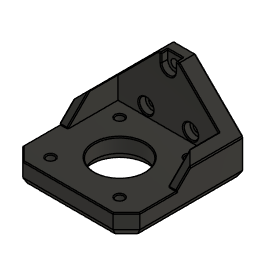
z_axis_bottom_x2 (Autodesk Fusion 360 design; units mm, degrees)
Autodesk Fusion 360 part; units mm, degrees
note: some values were not read from the file. Chosen so that the rebuilt part matches the saved one: which face or edge a step refers to; the sign of a taper; which pieces of a blend or face edit are solid. Set by a fixed rule: which sketch regions a step uses.
sketch "Sketch1" plane through (0, 0, 0) normal (0, 0, 1) x (1, 0, 0)
  line L0 (0, 0) -> (52.5, 0)
  line L1 (52.5, 0) -> (52.5, 52.5)
  line L2 (52.5, 52.5) -> (0, 52.5)
  line L3 (0, 52.5) -> (0, 0)
  line L4 (0, 6) -> (6, 0)
  line L5 (26.25, 0) -> (26.25, 50)
  line L6 (3.7, 22.5) -> (0, 22.5)
  line L7 (3.7, 45) -> (26.25, 45)
  line L8 (3.7, 22.5) -> (3.7, 45)
  circle A0 centre (26.25, 23.2) radius 11.2
  line L9 (48.8, 22.5) -> (52.5, 22.5)
  line L10 (48.8, 22.5) -> (48.8, 45)
  line L11 (48.8, 45) -> (26.25, 45)
  line L12 (52.5, 6) -> (46.5, 0)
  circle A1 centre (10.75, 38.7) radius 1.75
  line L13 (10.75, 38.7) -> (41.75, 7.7) construction
  line L14 (41.75, 38.7) -> (10.75, 7.7) construction
  line L15 (41.75, 38.7) -> (10.75, 38.7) construction
  line L16 (10.75, 38.7) -> (10.75, 7.7) construction
  circle A2 centre (10.75, 38.7) radius 3.25
  line L17 (9, 41.4386) -> (9, 35.9614)
  line L18 (12.5, 41.4386) -> (12.5, 35.9614)
  line L19 (9, 40.45) -> (12.5, 40.45)
  line L20 (12.5, 36.95) -> (9, 36.95)
  line L21 (26.25, 23.2) -> (10.75, 23.2)
  circle A3 centre (10.75, 7.7) radius 3.25
  line L22 (12.5, 9.45) -> (9, 9.45)
  line L23 (12.5, 4.9614) -> (12.5, 10.4386)
  circle A4 centre (10.75, 7.7) radius 1.75
  line L24 (9, 5.95) -> (12.5, 5.95)
  line L25 (9, 4.9614) -> (9, 10.4386)
  line L26 (40, 36.95) -> (43.5, 36.95)
  line L27 (40, 41.4386) -> (40, 35.9614)
  circle A5 centre (41.75, 38.7) radius 1.75
  line L28 (43.5, 40.45) -> (40, 40.45)
  circle A6 centre (41.75, 38.7) radius 3.25
  line L29 (43.5, 41.4386) -> (43.5, 35.9614)
  circle A7 centre (41.75, 7.7) radius 1.75
  line L30 (43.5, 5.95) -> (40, 5.95)
  line L31 (40, 9.45) -> (43.5, 9.45)
  line L32 (40, 4.9614) -> (40, 10.4386)
  line L33 (43.5, 4.9614) -> (43.5, 10.4386)
  circle A8 centre (41.75, 7.7) radius 3.25
  line L34 (3.7, 45) -> (0, 45)
  line L35 (48.8, 45) -> (52.5, 45)
  point P0 (26.25, 23.2)
  dimension "d1" = 52.5
  dimension "d3" = 45
  dimension "d6" = 6
  dimension "d7" = 3.7
  dimension "d8" = 7.5
  dimension "d9" = 22.5
  dimension "d10" = 22.4
  dimension "d11" = 23.2
  dimension "d12" = 3.5
  dimension "d13" = 90
  dimension "d14" = 31
  dimension "d15" = 6.5
  dimension "d65" = 52.5
  constraint horizontal L0
  constraint vertical L1
  constraint horizontal L2
  constraint vertical L3
  constraint coincident L0.start L3.end
  constraint coincident L3 L4.start
  constraint coincident L0 L4.end
  constraint midpoint L0 L5.start
  constraint coincident L3 L6.end
  constraint horizontal L6
  constraint coincident L5 L7.end
  constraint horizontal L7
  constraint vertical L8
  constraint coincident L7.start L8.end
  constraint coincident L5 P0
  constraint symmetric L5 L6.start L9.start
  constraint symmetric L5 L6.end L9.end
  constraint symmetric L5 L7.start L10.end
  constraint symmetric L5 L7.end L11.end
  constraint symmetric L4.start L5 L12.start
  constraint symmetric L4.end L5 L12.end
  constraint midpoint L13 P0
  constraint midpoint P0 L14
  constraint horizontal L15
  constraint coincident A1.centre L13.start
  constraint vertical L16
  constraint coincident L14.end L16.end
  constraint coincident P0 A0.centre
  constraint concentric A1 A2
  constraint coincident A2 L17.start
  constraint coincident A2 L17.end
  constraint coincident A2 L18.start
  constraint coincident A2 L18.end
  constraint vertical L18
  constraint vertical L17
  constraint tangent A1 L17
  constraint tangent A1 L18
  constraint coincident L17 L19.start
  constraint coincident L18 L19.end
  constraint coincident L18 L20.start
  constraint coincident L17 L20.end
  constraint horizontal L19
  constraint horizontal L20
  constraint tangent A1 L19
  constraint tangent A1 L20
  constraint midpoint L16 L21.end
  constraint symmetric A1 L21 A4
  constraint symmetric A2 L21 A3
  constraint symmetric L17.start L21 L25.start
  constraint symmetric L17.end L21 L25.end
  constraint symmetric L18.start L21 L23.start
  constraint symmetric L18.end L21 L23.end
  constraint symmetric L19.start L21 L24.start
  constraint symmetric L19.end L21 L24.end
  constraint symmetric L20.start L21 L22.start
  constraint symmetric L20.end L21 L22.end
  constraint symmetric L5 A1 A5
  constraint symmetric L5 A2 A6
  constraint symmetric L5 L17.start L29.start
  constraint symmetric L5 L17.end L29.end
  constraint symmetric L5 L18.start L27.start
  constraint symmetric L5 L18.end L27.end
  constraint symmetric L5 L19.start L28.start
  constraint symmetric L5 L19.end L28.end
  constraint symmetric L5 L20.start L26.start
  constraint symmetric L5 L20.end L26.end
  constraint vertical L5
  constraint symmetric L5 A3 A8
  constraint symmetric L5 L22.start L31.start
  constraint symmetric L5 L22.end L31.end
  constraint symmetric L5 L23.start L32.start
  constraint symmetric L5 L23.end L32.end
  constraint symmetric L5 A4 A7
  constraint symmetric L5 L24.start L30.start
  constraint symmetric L5 L24.end L30.end
  constraint symmetric L5 L25.start L33.start
  constraint symmetric L5 L25.end L33.end
  constraint coincident L3 L34.end
  constraint perpendicular L3 L34
  constraint symmetric L5 L34.end L35.end
  measures "d1" distance of L0.start L0.end
  measures "d3" angle of L0 L4
  measures "d6" distance of L0.start L4.end
  measures "d7" distance of L6.start L6.end
  measures "d8" distance of L2 L7
  measures "d9" distance of L6.start L7.start
  measures "d10" diameter of A0
  measures "d11" distance of L5.start P0
  measures "d12" diameter of A1
  measures "d13" angle of L13 L14
  measures "d14" distance of L14.start A1.centre
  measures "d15" diameter of A2
  measures "d65" distance of L0.start L2.end
extrude "Extrude1" add sketch "Sketch1" along normal blind 9 contours L0 L3 L4 L5 L6 L7 L8 A0 | L0 L1 L5 A0 L9 L10 L11 L12 | L3 L6 L8 L34 | L1 L9 L10 L35 | A1 L18 L20 | A1 L18 L19 | A2 L18 | A1 L17 L19 | A2 L17 L18 L19 | A1 L17 L20 | A2 L17 L18 L20 | A2 L17 | A3 L23 | A3 L22 L23 L25 | A3 L23 L24 L25 | A3 L25 | L22 L23 A4 | L23 A4 L24 | L22 A4 L25 | A4 L24 L25 | L26 L27 A5 | L26 L27 A6 L29 | L27 A6 | L26 A5 L29 | L27 A5 L28 | A6 L29 | A5 L28 L29 | L27 L28 A6 L29 | A7 L30 L33 | L33 A8 | A7 L31 L33 | A7 L31 L32 | L31 L32 L33 A8 | A7 L30 L32 | L30 L32 L33 A8 | L32 A8
extrude "Extrude2" cut sketch "Sketch1" along normal blind 3.6 contours A1 L18 L20 | A1 L18 L19 | A1 L17 L19 | A1 L17 L20 | L22 L23 A4 | L23 A4 L24 | L22 A4 L25 | A4 L24 L25 | L26 L27 A5 | L26 A5 L29 | L27 A5 L28 | A5 L28 L29 | A7 L30 L33 | A7 L31 L33 | A7 L31 L32 | A7 L30 L32
extrude "Extrude3" cut sketch "Sketch1" along normal blind 3.3 contours A2 L17 L18 L19 | A2 L17 L18 L20 | A3 L22 L23 L25 | A3 L23 L24 L25 | L26 L27 A6 L29 | L27 L28 A6 L29 | L31 L32 L33 A8 | L30 L32 L33 A8
extrude "Extrude4" cut sketch "Sketch1" along normal blind 3 contours A2 L18 | A2 L17 | A3 L23 | A3 L25 | L27 A6 | A6 L29 | L33 A8 | L32 A8
extrude "Extrude6" add sketch "Sketch1" along normal blind 37 contours L1 L2 L3 L7 L11 L34 L35
extrude "Extrude7" add sketch "Sketch1" along normal blind 32 contours L3 L6 L8 L34 | L1 L9 L10 L35
chamfer "Chamfer3" distance 22.5 angle 45 2 edges at (50.65, 22.5, 32) (1.85, 22.5, 32) measured on face at (50.0333, 37.5, 32) measured on face at (1.2333, 37.5, 32)
chamfer "Chamfer4" distance 21.5 angle 45 2 edges at (52.5, 48.75, 37) (0, 48.75, 37) measured on face at (17.5, 50, 37) measured on face at (17.5, 50, 37)
chamfer "Chamfer6" distance 1.5 angle 60 6 edges at (52.5, 29.25, 0) (49.5, 3, 0) (26.25, 0, 0) (3, 3, 0) (0, 29.25, 0) (26.25, 52.5, 0) measured on face at (30.9178, 48.8616, 0) measured on face at (50.5, 4, 3) measured on face at (30.9178, 48.8616, 0) measured on face at (30.9178, 48.8616, 0) measured on face at (30.9178, 48.8616, 0) measured on face at (30.9178, 48.8616, 0)
chamfer "Chamfer7" distance 0.4 angle 45 9 edges at (38.7199, 6.5247, 0) (7.7199, 6.5247, 0) (7.7199, 37.5247, 0) (38.7199, 37.5247, 0) (9.1184, 39.3328, 9) (9.1184, 8.3328, 9) (40.1184, 8.3328, 9) (40.1184, 39.3328, 9) (15.8079, 27.2501, 9) measured on face at (30.9178, 47.8616, 0) measured on face at (30.9178, 47.8616, 0) measured on face at (30.9178, 47.8616, 0) measured on face at (30.9178, 47.8616, 0) measured on face at (42.6306, 28.665, 9) measured on face at (42.6306, 28.665, 9) measured on face at (42.6306, 28.665, 9) measured on face at (42.6306, 28.665, 9) measured on face at (42.6306, 28.665, 9)
chamfer "Chamfer8" distance 1.5 angle 60 1 edges at (15.8079, 19.1499, 0) measured on face at (21.5783, 48.0114, 0)
sketch "Sketch2" plane through (0, 45, 0) normal (0, -1, 0) x (1, 0, 0)
  line L0 (21.5, 37) -> (3.7, 19.2) construction
  line L1 (3.7, 19.2) -> (3.7, 9) construction
  line L2 (3.7, 9) -> (48.8, 9) construction
  line L3 (48.8, 9) -> (48.8, 19.2) construction
  line L4 (48.8, 19.2) -> (31, 37) construction
  line L5 (31, 37) -> (21.5, 37)
  line L6 (26.25, 37) -> (26.25, 9)
  line L7 (3.7, 9) -> (3.7, 0) construction
  line L8 (3.7, 0) -> (48.8, 0) construction
  line L9 (48.8, 0) -> (48.8, 9) construction
  circle A0 centre (16.25, 13) radius 3.25
  circle A1 centre (16.25, 13) radius 1.75
  circle A2 centre (36.25, 13) radius 3.25
  circle A3 centre (36.25, 13) radius 1.75
  circle A4 centre (26.25, 33) radius 3.25
  circle A5 centre (26.25, 33) radius 1.75
  line L10 (23, 33) -> (23, 37)
  line L11 (29.5, 33) -> (29.5, 37)
  line L12 (36.25, 13) -> (16.25, 13) construction
  line L13 (20.25, 8.52) -> (32.25, 8.52)
  line L14 (32.25, 8.52) -> (32.25, 17.48)
  line L15 (32.25, 17.48) -> (20.25, 17.48)
  line L16 (20.25, 17.48) -> (20.25, 8.52)
  line L17 (20.25, 8.52) -> (32.25, 17.48) construction
  line L18 (32.25, 8.52) -> (20.25, 17.48) construction
  line L19 (36.25, 13) -> (46.5, 13) construction
  line L20 (40.25, 8.52) -> (47.5, 8.52)
  line L21 (47.5, 8.52) -> (47.5, 17.48)
  line L22 (47.5, 17.48) -> (40.25, 17.48)
  line L23 (40.25, 17.48) -> (40.25, 8.52)
  line L24 (40.25, 8.52) -> (47.5, 17.48) construction
  line L25 (47.5, 8.52) -> (40.25, 17.48) construction
  line L26 (5, 8.52) -> (5, 17.48)
  line L27 (5, 17.48) -> (12.25, 17.48)
  line L28 (12.25, 17.48) -> (12.25, 8.52)
  line L29 (12.25, 8.52) -> (5, 8.52)
  line L30 (52.5, 2.5981) -> (52.5, 15.5)
  point P0 (26.25, 13)
  point P1 (43.875, 13)
  dimension "d49" = 9
  dimension "d50" = 6.5
  dimension "d51" = 3.5
  dimension "d52" = 20
  dimension "d53" = 13
  dimension "d54" = 6.5
  dimension "d55" = 3.5
  dimension "d56" = 33
  dimension "d68" = 8.96
  dimension "d69" = 4
  dimension "d71" = 8.96
  dimension "d72" = 4
  dimension "d91" = 5
  constraint midpoint L5 L6.start
  constraint midpoint L2 L6.end
  constraint coincident L1.end L2.start
  constraint perpendicular L2 L7
  constraint perpendicular L7 L8
  constraint perpendicular L8 L9
  constraint coincident L2.end L3.start
  constraint concentric A0 A1
  constraint symmetric L6 A0 A2
  constraint symmetric L6 A1 A3
  constraint coincident L6 A4.centre
  constraint concentric A4 A5
  constraint coincident A4 L10.start
  constraint tangent A4 L10
  constraint coincident L5 L10.end
  constraint coincident A4 L11.start
  constraint tangent A4 L11
  constraint coincident L5 L11.end
  constraint vertical L11
  constraint vertical L10
  constraint coincident A2.centre A3.centre
  constraint coincident A0.centre A1.centre
  constraint horizontal L13
  constraint perpendicular L13 L14
  constraint parallel L13 L15
  constraint parallel L14 L16
  constraint coincident L17 P0
  constraint coincident L18 P0
  constraint midpoint L12 P0
  constraint perpendicular L3 L19
  constraint horizontal L20
  constraint perpendicular L20 L21
  constraint parallel L20 L22
  constraint parallel L21 L23
  constraint coincident L24 P1
  constraint coincident L25 P1
  constraint coincident L19 P1
  constraint symmetric L6 L20.start L28.end
  constraint symmetric L6 L20.end L26.start
  constraint symmetric L6 L21.end L26.end
  constraint symmetric L6 L22.end L27.end
  measures "d49" distance of L8.end L2.end
  measures "d50" diameter of A0
  measures "d51" diameter of A1
  measures "d53" distance of L8 A0.centre
  measures "d54" diameter of A4
  measures "d55" diameter of A5
  measures "d56" distance of L8 A4.centre
  measures "d68" distance of L13.end L14.end
  measures "d69" distance of A0.centre L16
  measures "d71" distance of L20.end L21.end
  measures "d72" distance of A2.centre L23
  measures "d91" distance of L21 L30
extrude "Extrude8" cut sketch "Sketch2" against normal blind 7.5 contours L6 A5 | L6 A5 | A1 | A3
extrude "Extrude9" cut sketch "Sketch2" against normal blind 3 contours L5 L6 A4 L11 | L5 L6 A4 L10 | L6 A4 A5 | L6 A4 A5 | A0 | A2
chamfer "Chamfer9" distance 0.4 angle 45 30 edges at (52.5, 14.25, 9) (49.5, 3, 9) (26.25, 0, 9) (3, 3, 9) (0, 14.25, 9) (12.6, 45, 28.1) (22.25, 45, 37) (23, 45, 35) (26.25, 45, 29.75) (29.5, 45, 35) (30.25, 45, 37) (39.9, 45, 28.1) (33, 45, 13) (13, 45, 13) (48.8, 27.3478, 14.3523) (48.8, 22.5, 9.2523) (48.8, 38.5978, 19.2) (52.5, 22.5, 9.2523) (52.5, 40.4977, 15.5) (52.5, 25.4977, 12.5023) (0, 22.5, 9.2523) (0, 25.4977, 12.5023) (0, 40.4977, 15.5) (3.7, 22.5, 9.2523) (3.7, 27.3477, 14.3523) (3.7, 38.5977, 19.2) (24.5, 52.5, 33) (34.5, 52.5, 13) (14.5, 52.5, 13) (26.25, 48, 37)
chamfer "Chamfer10" distance 0.4 angle 45 2 edges at (29.5, 46.9, 37) (23, 46.9, 37) measured on face at (27.3333, 51.1333, 37) measured on face at (27.3333, 51.1333, 37)
extrude "Extrude10" add sketch "Sketch2" against normal blind 1.4 from surface at -7.5 contours L13 L14 L15 L16 | L20 L21 L22 L23 | L26 L27 L28 L29
fillet "Fillet1" radius 1.4 6 edges at (47.5, 53.9, 13) (40.25, 53.9, 13) (32.25, 53.9, 13) (20.25, 53.9, 13) (12.25, 53.9, 13) (5, 53.9, 13)
draft "Draft1" angle 50 neutral plane through (52.5, 52.5, 0) pull (0, 1, 0) 1 faces at (43.1332, 52.9667, 8.52)
draft "Draft2" angle -50 neutral plane through (52.5, 52.5, 0) pull (0, -1, 0) 1 faces at (24.7166, 52.9667, 8.52)
draft "Draft3" angle -50 neutral plane through (52.5, 52.5, 0) pull (0, -1, 0) 1 faces at (7.8832, 52.9667, 8.52)
draft "Draft4" angle -50 neutral plane through (52.5, 52.5, 0) pull (0, -1, 0) 1 faces at (7.8832, 52.9667, 17.48)
draft "Draft5" angle -50 neutral plane through (52.5, 52.5, 0) pull (0, -1, 0) 1 faces at (24.7166, 52.9667, 17.48)
draft "Draft6" angle -50 neutral plane through (52.5, 52.5, 0) pull (0, -1, 0) 1 faces at (43.1332, 52.9667, 17.48)
chamfer "Chamfer12" distance 0.4 angle 45 7 edges at (41.6086, 52.5, 26.3914) (26.25, 52.5, 37) (10.8914, 52.5, 26.3914) (52.3586, 52.5, 15.4414) (0.1414, 52.5, 15.4414) (0, 52.5, 8.849) (52.5, 52.5, 8.849) measured on face at (44.1, 50.1333, 23.9) measured on face at (27.4667, 51.1333, 37) measured on face at (8.4, 50.1333, 23.9) measured on face at (52.4057, 36.7017, 15.3276) measured on face at (0.0943, 36.7017, 15.3276) measured on face at (26.3036, 52.5, 21.9387) measured on face at (52.5, 44.5537, 10.9327)
equation "d11 = ( ( 22.4 / 2 ) * 1 mm ) + 9.5 mm + 2.5 mm"
equation "d30 = 9 mm + 28 mm"
equation "d32 = 9 mm + 23 mm"
equation "d40 = chamfer_bed"
equation "d41 = corner_angle_bed"
equation "chamfer_bed = 1.5 mm"
equation "corner_angle_bed = 60 deg"
equation "chamfer_small = 0.4 mm"
equation "d45 = chamfer_small"
equation "d47 = chamfer_bed"
equation "d48 = corner_angle_bed"
equation "d56 = 13 mm + 20 mm"
equation "d61 = chamfer_small"
equation "d63 = chamfer_small"
equation "d92 = chamfer_small"
